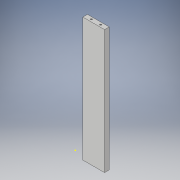
# Autodesk Inventor part: LeftSideTopPlateConnector
Saved by Autodesk Inventor 2017 (Build 210142000, 142)
## iProperties
Created: 2017-12-13
Part Number: LeftSideTopPlateConnector
Material: Generic
Document SubType Name: Modeling
Designer: User
Density: 1 g/cm^3
Appearance: Default
Author: User
Autodesk Inventor part; units mm, degrees
ref_plane "YZ Plane" through (0, 0, 0) normal (1, 0, 0) x (0, 1, 0)
ref_plane "XZ Plane" through (0, 0, 0) normal (0, 1, 0) x (-1, 0, 0)
ref_plane "XY Plane" through (0, 0, 0) normal (0, 0, 1) x (1, 0, 0)
sketch "Sketch1" plane through (0, 0, 0) normal (0, 0, 1) x (1, 0, 0)
  line L0 (0, 0) -> (69.215, 0)
  line L1 (69.215, 0) -> (69.215, -254)
  line L2 (69.215, -254) -> (0, -254)
  line L3 (0, -254) -> (0, 0)
  dimension "d0" = 69.215
  dimension "d1" = 254
  constraints: 8 end point, 2 parallel, 1 horizontal, 1 perpendicular
  measures "d0" distance of L1.end L2.end
  measures "d1" distance of L0.end L1.end
extrude "Extrusion1" add sketch "Sketch1" along normal blind 9.525
sketch "Sketch4" plane through (0, 0, 0) normal (0, 0, -1) x (-1, 0, 0)
  line L0 (-69.215, -254) -> (0, -254) projected
  line L1 (0, 0) -> (-24.765, 0)
  line L2 (-24.765, 0) -> (-24.765, -254)
  line L3 (-24.765, -254) -> (0, -254)
  line L4 (0, -254) -> (0, 0)
  dimension "d11" = 24.765
  constraints: 8 end point, 2 parallel, 1 horizontal, 1 perpendicular, 1 point on line
  measures "d11" distance of L3.end L2.end
extrude "Extrusion4" cut sketch "Sketch4" against normal blind 127
sketch "Sketch5" plane through (69.215, -254, 0) normal (0, -1, 0) x (1, 0, 0)
  point P0 (-69.215, 0)
sketch "Sketch8" plane through (69.215, 0, 9.525) normal (0, 1, 0) x (1, 0, 0)
  line L0 (-44.45, 0) -> (-44.45, 9.525) projected
  line L1 (0, 9.525) -> (0, 0) projected
  point P0 (-69.215, 9.525)
  point P1 (-12.7, 4.7625)
  point P2 (-12.7, 4.7625)
  point P3 (-31.75, 4.7625)
hole "Hole1" at (37.465, 0, 4.7625) at (56.515, 0, 4.7625) direction (0, -1, 0) diameter 3.302 depth 7.62 tip angle 118 thread size "8-32 UNC" class "2B" standard "ANSI Unified Screw Threads"
sketch "Sketch9" plane through (69.215, -254, 0) normal (0, -1, 0) x (1, 0, 0)
  line L0 (-44.45, 9.525) -> (-44.45, 0) projected
  line L1 (0, 0) -> (0, 9.525) projected
  point P0 (-69.215, 0)
  point P1 (-12.7, 4.7625)
  point P2 (-31.75, 4.7625)
hole "Hole2" at (37.465, -254, 4.7625) at (56.515, -254, 4.7625) direction (0, 1, 0) diameter 3.302 depth 7.62 tip angle 118 thread size "8-32 UNC" class "2B" standard "ANSI Unified Screw Threads"
body "Solid1"
